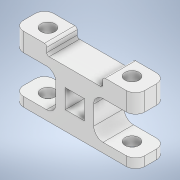
# Autodesk Inventor part: fuselage_CM904_interface
Saved by Autodesk Inventor 2021 (Build 250183000, 183)
## iProperties
Created: 2020-11-22
Part Number: fuselage_CM904_interface
Material: ABS Plastic
Document SubType Name: Modeling
Designer: Paco
Density: 1.06 g/cm^3
Appearance: Smooth - White
Mass: 0.647731 g
Surface Area: 7.58447 cm^2
Volume: 0.611067 cm^3
Author: Paco
Autodesk Inventor part; units mm, degrees
ref_plane "YZ Plane" through (0, 0, 0) normal (1, 0, 0) x (0, 1, 0)
ref_plane "XZ Plane" through (0, 0, 0) normal (0, 1, 0) x (-1, 0, 0)
ref_plane "XY Plane" through (0, 0, 0) normal (0, 0, 1) x (1, 0, 0)
sketch "Sketch1" plane through (0, 0, 0) normal (0, 0, 1) x (1, 0, 0)
  line L0 (2.05, 2.05) -> (-2.05, 2.05)
  line L1 (-2.05, 2.05) -> (-2.05, -2.05)
  line L2 (-2.05, -2.05) -> (2.05, -2.05)
  line L3 (2.05, -2.05) -> (2.05, 2.05)
  line L4 (2.05, 2.05) -> (-2.05, -2.05) construction
  line L5 (-2.05, 2.05) -> (2.05, -2.05) construction
  line L6 (4.05, 4.05) -> (-4.05, 4.05)
  line L7 (-4.05, 4.05) -> (-4.05, -4.05)
  line L8 (-4.05, -4.05) -> (4.05, -4.05)
  line L9 (4.05, -4.05) -> (4.05, 4.05)
  line L10 (4.05, 4.05) -> (-4.05, -4.05) construction
  line L11 (-4.05, 4.05) -> (4.05, -4.05) construction
  point P0 (0, 0)
  point P1 (0, 0)
  point P2 (0, 0)
  point P3 (0, 0)
  dimension "d24" = 8.1
  dimension "d25" = 4.1
  dimension "d26" = 8.1
  constraints: 24 end point, 6 midpoint, 4 parallel, 2 horizontal, 2 perpendicular, 1 coincident, 1 point on line, 1 other
  measures "d24" distance of L6.start L6.end
  measures "d25" distance of L0.start L0.end
  measures "d26" distance of L6.end L7.end
extrude "Extrusion1" add sketch "Sketch1" along normal blind 6.5
sketch "Sketch2" plane through (-5.0868, 4.05, 0) normal (0, 1, 0) x (1, 0, 0)
  circle A0 centre (14.0868, -3.25) radius 1.5
  circle A1 centre (-3.9132, -3.25) radius 1.5
  line L0 (12, 0) -> (0, 0) projected
  line L1 (12, -6.5) -> (0, -6.5) projected
  line L2 (-7.9132, -6.5) -> (18.0868, -6.5)
  line L3 (18.0868, -6.5) -> (18.0868, 0)
  line L4 (18.0868, 0) -> (-7.9132, 0)
  line L5 (-7.9132, 0) -> (-7.9132, -6.5)
  line L6 (5.0868, -6.5) -> (5.0868, 0) construction
  line L7 (1.0368, 0) -> (1.0368, -6.5) projected
  line L8 (9.1368, 0) -> (9.1368, -6.5) projected
  point P0 (5.0868, 0)
  dimension "d8" = 3
  dimension "d9" = 3
  dimension "d10" = 18
  dimension "d11" = 6.5
  dimension "d14" = 4
  dimension "d15" = 4
  dimension "d16" = 3.25
  dimension "d17" = 3.25
  dimension "d18" = 0
  dimension "d23" = 3.25
  dimension "d30" = 26
  dimension "d31" = 8.1
  dimension "d32" = 8.95
  constraints: 10 end point, 2 centre point, 2 midpoint, 2 parallel, 1 horizontal, 1 perpendicular
  measures "d8" diameter of A0
  measures "d9" diameter of A1
  measures "d10" distance of A1.centre A0.centre
  measures "d11" distance between parallel lines of L0 L1
  measures "d14" distance from line of L5 A1.centre
  measures "d15" distance from line of L3 A0.centre
  measures "d16" distance from line of L4 A1.centre
  measures "d17" distance from line of L2 A1.centre
  measures "d18" distance between parallel lines of L0 L4
  measures "d23" distance from line of L2 A0.centre
  measures "d30" distance between parallel lines of L3 L5
  measures "d31" distance between parallel lines of L8 L7
  measures "d32" distance between parallel lines of L7 L5
extrude "Extrusion2" add sketch "Sketch2" along normal blind 4
fillet "Fillet1" radius 2 2 edges at (4.05, 4.05, 3.25) (-4.05, 4.05, 3.25)
fillet "Fillet2" radius 2 2 edges at (-4.05, -4.05, 3.25) (4.05, -4.05, 3.25)
fillet "Fillet3" radius 2 4 edges at (-13, 6.05, 6.5) (13, 6.05, 6.5) (13, 6.05, 0) (-13, 6.05, 0)
sketch "Sketch3" plane through (-5.0868, 8.05, 0) normal (0, 1, 0) x (1, 0, 0)
  line L0 (-5.9132, -6.5) -> (16.0868, -6.5) projected
  line L1 (16.0868, 0) -> (-5.9132, 0) projected
  line L2 (11.0868, -6.5) -> (-0.9132, -6.5)
  line L3 (-0.9132, -6.5) -> (-0.9132, 0)
  line L4 (-0.9132, 0) -> (11.0868, 0)
  line L5 (11.0868, 0) -> (11.0868, -6.5)
  line L6 (-7.9132, -2) -> (-7.9132, -4.5) projected
  line L7 (18.0868, -4.5) -> (18.0868, -2) projected
  point P0 (5.0868, 0)
  point P1 (11.0868, 0)
  point P2 (-0.9132, -6.5)
  dimension "d33" = 7
  dimension "d34" = 7
  constraints: 8 end point, 2 parallel, 2 point on line, 1 horizontal, 1 perpendicular
  measures "d33" distance between parallel lines of L3 L6
  measures "d34" distance between parallel lines of L7 L5
extrude "Extrusion3" cut sketch "Sketch3" against normal blind 2
fillet "Fillet4" radius 0.5 4 edges at (6, 8.05, 3.25) (-6, 8.05, 3.25) (-6, 6.05, 3.25) (6, 6.05, 3.25)
mirror "Mirror1" about plane through (0, 0, 0) normal (0, 1, 0)
sketch "Sketch5" plane through (6.5, -8.05, 0) normal (0, -1, 0) x (1, 0, 0)
  line L0 (12.0758, -8.2102) -> (-27.8852, -8.2102)
  line L1 (-27.8852, -8.2102) -> (-27.8852, 11.7461)
  line L2 (-27.8852, 11.7461) -> (12.0758, 11.7461)
  line L3 (12.0758, 11.7461) -> (12.0758, -8.2102)
  point P0 (-6.5, 0)
  constraints: 8 end point, 2 parallel, 1 horizontal, 1 perpendicular
extrude "Extrusion4" cut sketch "Sketch5" against normal up to surface (2 mm away)
equation "\"d16\" = d17"
equation "\"d23\" = d17"
equation "\"d32\" = -0.5 * d31 + 0.5 * d30"
body "Solid1"
